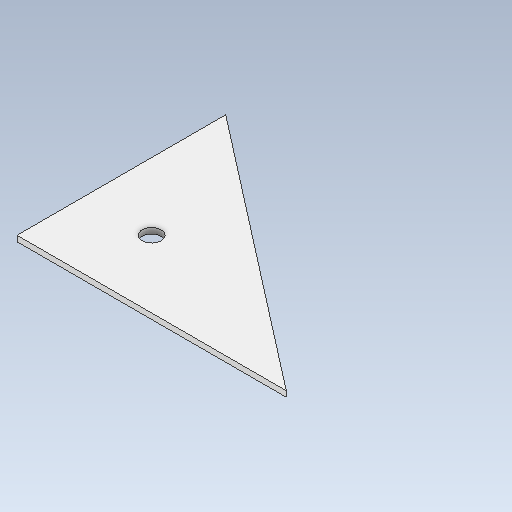
# Autodesk Inventor part: Base_Ruedas
Saved by Autodesk Inventor 2021 (Build 250183000, 183)
## iProperties
Created: 2021-05-06
Part Number: Base_Ruedas
Material: Acero ASTM A36
Document SubType Name: Chapa
Designer: Admin
Density: 7.85 g/cm^3
Sheet Metal Rule: Default_mm
Appearance: Placa
Mass: 108.394 g
Surface Area: 120.253 cm^2
Volume: 13.8081 cm^3
Flat Pattern Width: 7.35086 cm
Flat Pattern Length: 15.1819 cm
Flat Pattern Area: 111.6 cm^2
Sheet Metal Width: 73,509 mm
Sheet Metal Length: 151,819 mm
Sheet Metal Area: 11160,000 mm^2
Author: Admin
Autodesk Inventor part; units mm, degrees
ref_plane "YZ Plane" through (0, 0, 0) normal (1, 0, 0) x (0, 1, 0)
ref_plane "XZ Plane" through (0, 0, 0) normal (0, 1, 0) x (-1, 0, 0)
ref_plane "XY Plane" through (0, 0, 0) normal (0, 0, 1) x (1, 0, 0)
sketch "Boceto1" plane through (0, 0, 0) normal (0, 1, 0) x (-1, 0, 0)
  line L0 (0, 0) -> (-120, 0)
  line L1 (0, 0) -> (0, -93)
  line L2 (-120, 0) -> (0, -93)
  dimension "d0" = 120
  dimension "d1" = 93
  measures "d0" distance of L0.start L0.end
  measures "d1" distance of L0.start L1.end
extrude "Placa1" add sketch "Boceto1" along normal blind 2.5
sketch "Sketch2" plane through (0, 0, 0) normal (0, -1, 0) x (1, 0, 0)
  line L0 (0, 0) -> (120, 0) projected
  line L1 (0, -93) -> (0, 0) projected
  point P0 (30, -30)
  dimension "d3" = 30
  dimension "d4" = 30
  measures "d3" distance from line of L0 point (30, -30)
  measures "d4" distance from line of point (30, -30) L1
hole "Hole1" at (30, 0, -30) direction (0, 1, 0) diameter 8.5 depth 2.5 tip angle 118
thread "Thread1" size "M10x1.5" class "6H" standard "ISO Metric profile" full length
equation "\"d10\" = Grosor"
equation "\"d2\" = Grosor"
equation "\"Radio_pliegue\" = Grosor"
equation "\"Anchura_desahogo_plegado\" = Grosor"
equation "\"Profundidad_desahogo_plegado\" = 0.5 * Grosor"
equation "\"Remanente_mínimo\" = 2 * Grosor"
equation "\"Radiodetransición\" = Radio_pliegue"
equation "\"Tamaño_de_radio_de_Jacobi\" = Radio_pliegue"
equation "\"TamañoSeparación\" = Grosor"
equation "\"Grosor\" = 2.5"
